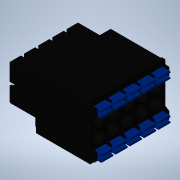
# Autodesk Inventor part: 8079510 10GD-2RR3,5-CLP-CBL
Saved by Autodesk Inventor 2021 (Build 250183000, 183)
## iProperties
Created: 2026-04-23
Part Number: 8079510 10GD-2RR3,5-CLP-CBL
Material: Generic
Catalog Web Link: www.3dfindit.com
Description: NEKM-C6 (p)-terminal strip
Vendor: FESTO
Document SubType Name: Modeling
Designer: psAdmin
Manufacturer: FESTO
Mass: 3.84274 g
Surface Area: 29.1557 cm^2
Volume: 3.84274 cm^3
Density: 1 g/cm^3
Appearance: PSOLRGB-80-80-80
Category: PARTsolutions
Company: FESTO
Title: 8079510 10GD-2RR3,5-CLP-CBL
Author: Cadenas PARTsolutions
Comments: terminal strip
PSOL_IDENT_0: {$CADENAS_DATA/23d-libs/festo/parts/n/nekm/parts/nekm_c6_parts.prj},200 {VTYP=3D},{NB=8079510 10GD-2
PSOL_IDENT_1: RR3,5-CLP-CBL},{LINA=8079510 10GD-2RR3,5-CLP-CBL},{NN=NEKM-C6 (p)},{DATE=26.08.2025 07:05:50},{GEOMD
PSOL_IDENT_2: ATE=26.08.2025 07:05:00},{VERSION=},{LINEID=160},{WBVAR=},{WBNUMERIC=}  {NB=8079510 10GD-2RR3,5-CLP-
PSOL_IDENT_3: CBL},{LINA=8079510 10GD-2RR3,5-CLP-CBL},{KT=DUMMY},{TNR=8079510},{TYP=10GD-2RR3,5-CLP-CBL},{VERS=1},
PSOL_IDENT_4: {N=5},{L=18.300},{L1=0.000}
NB: 8079510 10GD-2RR3,5-CLP-CBL
NN: NEKM-C6 (p)
NT: terminal strip
NBSYN: $TNR. $TYP.
LINA: 8079510 10GD-2RR3,5-CLP-CBL
CATALOG: Festo
TNR: 8079510
TYP: 10GD-2RR3,5-CLP-CBL
VERS: 1
N: 5
L: 18.3
L1: 0
SUPPLIER: FESTO
ARTICLENO: 8079510 10GD-2RR3,5-CLP-CBL
BOMINFO: 8079510 10GD-2RR3,5-CLP-CBL
CREATOR: CADENAS GmbH
Autodesk Inventor part; units mm, degrees
sketch "Sketch_1" plane through (0, 0, 0) normal (0, 0, 1) x (1, 0, 0)
  line L0 (0, -4.9505) -> (0.2, -5.5)
  line L1 (0.2, -5.5) -> (0.2, -6.5)
  line L2 (0.2, -6.5) -> (13.4, -6.5)
  arc A0 (13.4, -6.5) -> (13.6, -6.3) centre (13.4, -6.3) ccw
  line L3 (13.6, -6.3) -> (13.6, 6.55)
  arc A1 (13.6, 6.55) -> (13.4, 6.75) centre (13.4, 6.55) ccw
  line L4 (13.4, 6.75) -> (12.8, 6.75)
  arc A2 (12.8, 6.75) -> (12.6, 6.55) centre (12.8, 6.55) ccw
  line L5 (12.6, 6.55) -> (12.6, 6.5)
  line L6 (12.6, 6.5) -> (0.2, 6.5)
  line L7 (0.2, 6.5) -> (0.2, 5.5)
  line L8 (0.2, 5.5) -> (0, 4.9505)
  line L9 (0, 4.9505) -> (0, -4.9505)
  constraints: 20 end point, 6 point on circle, 3 centre point
extrude "Extrusion1" add sketch "Sketch_1" along normal mid plane 18.3
sketch "Sketch_2" plane through (0, 0, 9.15) normal (0, 0, 1) x (1, 0, 0)
  line L0 (13.6, 5.85) -> (13.6, 3.0572)
  arc A0 (13.7, 3.2304) -> (13.6, 3.0572) centre (13.8, 3.0572) ccw
  line L1 (13.7, 3.2304) -> (14.5, 3.6923)
  arc A1 (14.5, 3.6923) -> (14.6, 3.8655) centre (14.4, 3.8655) ccw
  line L2 (14.6, 3.8655) -> (14.6, 5.45)
  arc A2 (14.6, 5.45) -> (14.4, 5.65) centre (14.4, 5.45) ccw
  line L3 (14.4, 5.65) -> (13.8, 5.65)
  arc A3 (13.6, 5.85) -> (13.8, 5.65) centre (13.8, 5.85) ccw
  constraints: 8 end point, 8 point on circle, 4 centre point
extrude "Extrusion2" add sketch "Sketch_2" against normal blind 0.625
sketch "Sketch_3" plane through (0, 0, 9.15) normal (0, 0, 1) x (1, 0, 0)
  arc A0 (13.8, -5.65) -> (13.6, -5.85) centre (13.8, -5.85) ccw
  line L0 (13.8, -5.65) -> (14.4, -5.65)
  arc A1 (14.4, -5.65) -> (14.6, -5.45) centre (14.4, -5.45) ccw
  line L1 (14.6, -5.45) -> (14.6, -3.8655)
  arc A2 (14.6, -3.8655) -> (14.5, -3.6923) centre (14.4, -3.8655) ccw
  line L2 (14.5, -3.6923) -> (13.7, -3.2304)
  arc A3 (13.6, -3.0572) -> (13.7, -3.2304) centre (13.8, -3.0572) ccw
  line L3 (13.6, -3.0572) -> (13.6, -5.85)
  constraints: 8 end point, 8 point on circle, 4 centre point
extrude "Extrusion3" add sketch "Sketch_3" against normal blind 0.625
pattern_linear "Rectangular Pattern1" count 2 spacing 17.675 along (0, 0, -1) of "Extrusion2"
pattern_linear "Rectangular Pattern2" count 2 spacing 17.675 along (0, 0, -1) of "Extrusion3"
sketch "Sketch_8" plane through (0, 0, 5.475) normal (0, 0, 1) x (1, 0, 0)
  line L0 (13.6, 5.85) -> (13.6, 3.0572)
  arc A0 (13.7, 3.2304) -> (13.6, 3.0572) centre (13.8, 3.0572) ccw
  line L1 (13.7, 3.2304) -> (14.5, 3.6923)
  arc A1 (14.5, 3.6923) -> (14.6, 3.8655) centre (14.4, 3.8655) ccw
  line L2 (14.6, 3.8655) -> (14.6, 5.45)
  arc A2 (14.6, 5.45) -> (14.4, 5.65) centre (14.4, 5.45) ccw
  line L3 (14.4, 5.65) -> (13.8, 5.65)
  arc A3 (13.6, 5.85) -> (13.8, 5.65) centre (13.8, 5.85) ccw
  constraints: 8 end point, 8 point on circle, 4 centre point
extrude "Extrusion4" add sketch "Sketch_8" against normal blind 0.45
pattern_linear "Rectangular Pattern3" count 4 spacing 3.5 along (0, 0, -1) of "Extrusion4"
sketch "Sketch_10" plane through (0, 0, 5.475) normal (0, 0, 1) x (1, 0, 0)
  arc A0 (13.8, -5.65) -> (13.6, -5.85) centre (13.8, -5.85) ccw
  line L0 (13.8, -5.65) -> (14.4, -5.65)
  arc A1 (14.4, -5.65) -> (14.6, -5.45) centre (14.4, -5.45) ccw
  line L1 (14.6, -5.45) -> (14.6, -3.8655)
  arc A2 (14.6, -3.8655) -> (14.5, -3.6923) centre (14.4, -3.8655) ccw
  line L2 (14.5, -3.6923) -> (13.7, -3.2304)
  arc A3 (13.6, -3.0572) -> (13.7, -3.2304) centre (13.8, -3.0572) ccw
  line L3 (13.6, -3.0572) -> (13.6, -5.85)
  constraints: 8 end point, 8 point on circle, 4 centre point
extrude "Extrusion5" add sketch "Sketch_10" against normal blind 0.45
pattern_linear "Rectangular Pattern4" count 4 spacing 3.5 along (0, 0, -1) of "Extrusion5"
sketch "Sketch_6" plane through (0, 0, 8.425) normal (0, 0, 1) x (1, 0, 0)
  line L0 (13.6, 3.85) -> (15.4, 3.85)
  arc A0 (15.4, 3.85) -> (15.6, 4.05) centre (15.4, 4.05) ccw
  line L1 (15.6, 4.05) -> (15.6, 4.0747)
  arc A1 (15.6, 4.0747) -> (15.4261, 4.273) centre (15.4, 4.0747) ccw
  line L2 (15.4261, 4.273) -> (14.4418, 4.4026)
  arc A2 (14.4418, 4.9974) -> (14.4418, 4.4026) centre (14.481, 4.7) ccw
  line L3 (14.4418, 4.9974) -> (15.4261, 5.127)
  arc A3 (15.4261, 5.127) -> (15.6, 5.3253) centre (15.4, 5.3253) ccw
  line L4 (15.6, 5.3253) -> (15.6, 5.35)
  arc A4 (15.6, 5.35) -> (15.4, 5.55) centre (15.4, 5.35) ccw
  line L5 (15.4, 5.55) -> (13.6, 5.55)
  line L6 (13.6, 5.55) -> (13.6, 3.85)
  constraints: 14 end point, 10 point on circle, 5 centre point
extrude "Extrusion6" add sketch "Sketch_6" against normal blind 2.85
pattern_linear "Rectangular Pattern5" count 5 spacing 3.5 along (0, 0, -1) count 2 spacing 9.4 along (0, -1, 0) of "Extrusion6"
sketch "Sketch_12" plane through (0, 1.8, 0) normal (0, 1, 0) x (1, 0, 0)
  line L0 (10.6, -7) -> (13.6, -7)
  line L1 (13.6, -7) -> (13.6, -8.7)
  arc A0 (13.6, -8.7) -> (13.4, -8.5) centre (13.4, -8.7) ccw
  line L2 (13.4, -8.5) -> (10.6, -8.5)
  line L3 (10.6, -8.5) -> (10.6, -7)
  line L4 (10.6, -7) -> (13.6, -7)
  constraints: 10 end point, 2 point on circle, 1 centre point
revolve "Revolution1" cut sketch "Sketch_12" angle 360 about axis through (10.6, 1.8, 7) along (-1, 0, 0)
pattern_linear "Rectangular Pattern6" count 5 spacing 3.5 along (0, 0, -1) count 2 spacing 3.6 along (0, -1, 0) of "Revolution1"
sketch "Sketch_14" plane through (0, 0, 0) normal (1, 0, 0) x (0, 1, 0)
  line L0 (0.4, 8.375) -> (0.4, 8.0338)
  arc A0 (0.4, 8.0338) -> (0.4586, 7.8924) centre (0.6, 8.0338) ccw
  line L1 (0.4586, 7.8924) -> (0.7278, 7.6232)
  arc A1 (0.8266, 7.277) -> (0.7278, 7.6232) centre (-0.8, 7) ccw
  line L2 (0.8266, 7.277) -> (0.6203, 7.0707)
  arc A2 (0.6203, 7.0707) -> (0.6203, 6.9293) centre (0.691, 7) ccw
  line L3 (0.6203, 6.9293) -> (0.8266, 6.723)
  arc A3 (0.7278, 6.3768) -> (0.8266, 6.723) centre (-0.8, 7) ccw
  line L4 (0.7278, 6.3768) -> (0.4586, 6.1076)
  arc A4 (0.4586, 6.1076) -> (0.4, 5.9662) centre (0.6, 5.9662) ccw
  line L5 (0.4, 5.9662) -> (0.4, 5.625)
  line L6 (0.4, 5.625) -> (4.6, 5.625)
  line L7 (4.6, 5.625) -> (4.6, 8.375)
  line L8 (4.6, 8.375) -> (0.4, 8.375)
  constraints: 18 end point, 10 point on circle, 5 centre point
extrude "Extrusion7" add sketch "Sketch_14" against normal blind 7.05
pattern_linear "Rectangular Pattern7" count 5 spacing 3.5 along (0, 0, -1) of "Extrusion7"
sketch "Sketch_16" plane through (0, 0, 0) normal (1, 0, 0) x (0, 1, 0)
  arc A0 (-3.6989, 8.375) -> (-4.6, 7.4739) centre (-3.6989, 7.4739) ccw
  line L0 (-4.6, 7.4739) -> (-4.6, 6.5261)
  arc A1 (-4.6, 6.5261) -> (-3.6989, 5.625) centre (-3.6989, 6.5261) ccw
  line L1 (-3.6989, 5.625) -> (-0.4, 5.625)
  line L2 (-0.4, 5.625) -> (-0.4, 5.9662)
  arc A2 (-0.4, 5.9662) -> (-0.4586, 6.1076) centre (-0.6, 5.9662) ccw
  line L3 (-0.4586, 6.1076) -> (-0.7278, 6.3768)
  arc A3 (-0.8266, 6.723) -> (-0.7278, 6.3768) centre (0.8, 7) ccw
  line L4 (-0.8266, 6.723) -> (-0.6203, 6.9293)
  arc A4 (-0.6203, 6.9293) -> (-0.6203, 7.0707) centre (-0.691, 7) ccw
  line L5 (-0.6203, 7.0707) -> (-0.8266, 7.277)
  arc A5 (-0.7278, 7.6232) -> (-0.8266, 7.277) centre (0.8, 7) ccw
  line L6 (-0.7278, 7.6232) -> (-0.4586, 7.8924)
  arc A6 (-0.4586, 7.8924) -> (-0.4, 8.0338) centre (-0.6, 8.0338) ccw
  line L7 (-0.4, 8.0338) -> (-0.4, 8.375)
  line L8 (-0.4, 8.375) -> (-3.6989, 8.375)
  constraints: 18 end point, 14 point on circle, 7 centre point
extrude "Extrusion8" add sketch "Sketch_16" against normal blind 7.05
pattern_linear "Rectangular Pattern8" count 5 spacing 3.5 along (0, 0, -1) of "Extrusion8"
sketch "Sketch_18" plane through (0, 2.75, 0) normal (0, 1, 0) x (1, 0, 0)
  line L0 (-6.05, -7) -> (-7.05, -7)
  line L1 (-7.05, -7) -> (-7.05, -6.2)
  line L2 (-7.05, -6.2) -> (-6.05, -6.2)
  line L3 (-6.05, -6.2) -> (-6.05, -7)
  line L4 (-6.05, -7) -> (-7.05, -7)
  constraints: 10 end point
revolve "Revolution2" cut sketch "Sketch_18" angle 360 about axis through (-6.05, 2.75, 7) along (1, 0, 0)
pattern_linear "Rectangular Pattern9" count 5 spacing 3.5 along (0, 0, -1) count 2 spacing 5.5 along (0, -1, 0) of "Revolution2"
ref_plane "ANBAU_XY" through (0, 0, 0) normal (0, 1, 0) x (1, 0, 0)
ref_plane "ANBAU_YZ" through (0, 0, 0) normal (1, 0, 0) x (0, 0, -1)
ref_plane "ANBAU_ZX" through (0, 0, 0) normal (0, 0, -1) x (0, 1, 0)
ref_plane "CP1_XY" through (0, 0, 0) normal (1, 0, 0) x (0, 0, -1)
ref_plane "CP1_YZ" through (0, 0, 0) normal (0, 0, -1) x (0, 1, 0)
ref_plane "CP1_ZX" through (0, 0, 0) normal (0, 1, 0) x (1, 0, 0)
ref_plane "ECP_1_XY" through (2.6, 1.8, 7) normal (1, 0, 0) x (0, 0, -1)
ref_plane "ECP_1_YZ" through (2.6, 1.8, 7) normal (0, 0, -1) x (0, 1, 0)
ref_plane "ECP_1_ZX" through (2.6, 1.8, 7) normal (0, 1, 0) x (1, 0, 0)
ref_plane "ECP_10_XY" through (2.6, -1.8, -7) normal (1, 0, 0) x (0, 0, -1)
ref_plane "ECP_10_YZ" through (2.6, -1.8, -7) normal (0, 0, -1) x (0, 1, 0)
ref_plane "ECP_10_ZX" through (2.6, -1.8, -7) normal (0, 1, 0) x (1, 0, 0)
ref_plane "ECP_2_XY" through (2.6, 1.8, 3.5) normal (1, 0, 0) x (0, 0, -1)
ref_plane "ECP_2_YZ" through (2.6, 1.8, 3.5) normal (0, 0, -1) x (0, 1, 0)
ref_plane "ECP_2_ZX" through (2.6, 1.8, 3.5) normal (0, 1, 0) x (1, 0, 0)
ref_plane "ECP_3_XY" through (2.6, 1.8, 0) normal (1, 0, 0) x (0, 0, -1)
ref_plane "ECP_3_YZ" through (2.6, 1.8, 0) normal (0, 0, -1) x (0, 1, 0)
ref_plane "ECP_3_ZX" through (2.6, 1.8, 0) normal (0, 1, 0) x (1, 0, 0)
ref_plane "ECP_4_XY" through (2.6, 1.8, -3.5) normal (1, 0, 0) x (0, 0, -1)
ref_plane "ECP_4_YZ" through (2.6, 1.8, -3.5) normal (0, 0, -1) x (0, 1, 0)
ref_plane "ECP_4_ZX" through (2.6, 1.8, -3.5) normal (0, 1, 0) x (1, 0, 0)
ref_plane "ECP_5_XY" through (2.6, 1.8, -7) normal (1, 0, 0) x (0, 0, -1)
ref_plane "ECP_5_YZ" through (2.6, 1.8, -7) normal (0, 0, -1) x (0, 1, 0)
ref_plane "ECP_5_ZX" through (2.6, 1.8, -7) normal (0, 1, 0) x (1, 0, 0)
ref_plane "ECP_6_XY" through (2.6, -1.8, 7) normal (1, 0, 0) x (0, 0, -1)
ref_plane "ECP_6_YZ" through (2.6, -1.8, 7) normal (0, 0, -1) x (0, 1, 0)
ref_plane "ECP_6_ZX" through (2.6, -1.8, 7) normal (0, 1, 0) x (1, 0, 0)
ref_plane "ECP_7_XY" through (2.6, -1.8, 3.5) normal (1, 0, 0) x (0, 0, -1)
ref_plane "ECP_7_YZ" through (2.6, -1.8, 3.5) normal (0, 0, -1) x (0, 1, 0)
ref_plane "ECP_7_ZX" through (2.6, -1.8, 3.5) normal (0, 1, 0) x (1, 0, 0)
ref_plane "ECP_8_XY" through (2.6, -1.8, 0) normal (1, 0, 0) x (0, 0, -1)
ref_plane "ECP_8_YZ" through (2.6, -1.8, 0) normal (0, 0, -1) x (0, 1, 0)
ref_plane "ECP_8_ZX" through (2.6, -1.8, 0) normal (0, 1, 0) x (1, 0, 0)
ref_plane "ECP_9_XY" through (2.6, -1.8, -3.5) normal (1, 0, 0) x (0, 0, -1)
ref_plane "ECP_9_YZ" through (2.6, -1.8, -3.5) normal (0, 0, -1) x (0, 1, 0)
ref_plane "ECP_9_ZX" through (2.6, -1.8, -3.5) normal (0, 1, 0) x (1, 0, 0)
ref_plane "MD_XY" through (-7.05, 2.75, 7) normal (-1, 0, 0) x (0, 0, -1)
ref_plane "MD_YZ" through (-7.05, 2.75, 7) normal (0, 0, -1) x (0, -1, 0)
ref_plane "MD_ZX" through (-7.05, 2.75, 7) normal (0, -1, 0) x (-1, 0, 0)
ref_plane "OP_XY" through (-7.05, 6.625, -9.15) normal (1, 0, 0) x (0, 0, 1)
ref_plane "OP_YZ" through (-7.05, 6.625, -9.15) normal (0, 0, 1) x (0, -1, 0)
ref_plane "OP_ZX" through (-7.05, 6.625, -9.15) normal (0, -1, 0) x (1, 0, 0)
body "Solid1"
